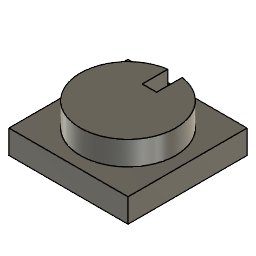
motorstand (Autodesk Fusion 360 design; units mm, degrees)
Autodesk Fusion 360 part; units mm, degrees
note: some values were not read from the file. Set by a fixed rule: which sketch regions a step uses.
sketch "Sketch1" plane through (0, 0, 0) normal (0, 0, 1) x (1, 0, 0)
  line L0 (0, 0) -> (-25, 0)
  line L1 (-25, 0) -> (-25, 25)
  line L2 (-25, 25) -> (0, 25)
  line L3 (0, 25) -> (0, 0)
  dimension "d1" = 25
  dimension "d2" = 25
  constraint horizontal L0
  constraint vertical L1
  constraint horizontal L2
  constraint vertical L3
  constraint coincident L0.start L3.end
  measures "d1" distance of L0.start L0.end
  measures "d2" distance of L0.start L2.end
extrude "Extrude1" add sketch "Sketch1" along normal blind 5
sketch "Sketch2" plane through (0, 0, 5) normal (0, 0, 1) x (-1, 0, 0)
  line L0 (0, -25) -> (25, -25)
  line L1 (25, -25) -> (25, 0)
  line L2 (25, 0) -> (0, 0)
  line L3 (0, 0) -> (0, -25)
  line L4 (12.5, -25) -> (12.5, 0)
  line L5 (12.5, -12.5) -> (0, -12.5)
  circle A0 centre (12.5, -12.5) radius 10
  dimension "d5" = 20
  constraint midpoint L0 L4.start
  constraint midpoint L2 L4.end
  constraint midpoint L4 L5.start
  constraint midpoint L3 L5.end
  constraint coincident L5.start A0.centre
  measures "d5" diameter of A0
extrude "Extrude2" add sketch "Sketch2" along normal blind 5 contours L4 L5 A0 | L4 A0 | L4 L5 A0
sketch "Sketch3" plane through (0, 0, 10) normal (0, 0, 1) x (-1, 0, 0)
  circle A0 centre (12.5, -12.5) radius 10
  line L0 (11, -17) -> (14, -17)
  line L1 (14, -17) -> (14, -23)
  line L2 (14, -23) -> (11, -23)
  line L3 (11, -23) -> (11, -17)
  constraint horizontal L0
  constraint vertical L1
  constraint horizontal L2
  constraint vertical L3
extrude "Extrude3" cut sketch "Sketch3" against normal blind 3 contours A0 L0 L1 L3 picked at (12.6672, -18.8291)
